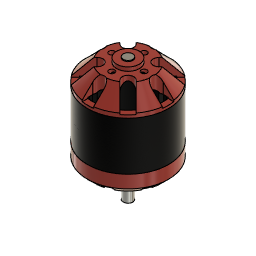
C4250-560KV (Autodesk Fusion 360 design; units mm, degrees)
Autodesk Fusion 360 part; units mm, degrees
sketch "Skizze1" plane through (0, 0, 0) normal (0, 0, 1) x (1, 0, 0)
  circle A0 centre (0, 0) radius 2.5
  dimension "d1" = 5
  constraint coincident A0.centre origin
  measures "d1" diameter of A0
extrude "Extrusion1" add sketch "Skizze1" against normal blind 0.5 makes body 1
sketch "Skizze2" plane through (0, 0, -0.5) normal (0, 0, -1) x (1, 0, 0)
  circle A0 centre (0, 0) radius 2.5
  circle A1 centre (0, 0) radius 5.95
  dimension "d4" = 11.9
  constraint coincident A0.centre A1.centre
  measures "d4" diameter of A1
extrude "Extrusion2" add sketch "Skizze2" along normal blind 2 separate body makes body 2
sketch "Skizze3" plane through (0, 0, -0.5) normal (0, 0, 1) x (-1, 0, 0)
  circle A0 centre (0, 0) radius 2.5
  circle A1 centre (0, 0) radius 5.95
sketch "Skizze4" plane through (0, 0, -2.5) normal (0, 0, -1) x (1, 0, 0)
  circle A0 centre (0, 0) radius 2.5
  circle A1 centre (0, 0) radius 5.95
  circle A2 centre (0, 0) radius 21.3
  dimension "d7" = 42.6
  constraint concentric A0 A2
  measures "d7" diameter of A2
extrude "Extrusion3" add sketch "Skizze4" along normal blind 46 separate body contours A2 makes body 3
sketch "Skizze5" plane through (0, 0, -2.5) normal (0, 0, 1) x (-1, 0, 0)
  circle A0 centre (0, 0) radius 5.95
  circle A1 centre (0, 0) radius 21.3
  circle A2 centre (0, 0) radius 12.75 construction
  dimension "d10" = 25.5
  constraint concentric A0 A2
  measures "d10" diameter of A2
chamfer "Fase1" distance 8.3 angle 45 1 edges at (-19.8586, 7.7024, -2.5) on bodies 3
sketch "Skizze6" plane through (0, 0, -2.5) normal (0, 0, 1) x (-1, 0, 0)
  circle A0 centre (8.5, 0) radius 1.5
  circle A1 centre (0, 8.5) radius 1.5
  circle A2 centre (-8.5, 0) radius 1.5
  circle A3 centre (0, -8.5) radius 1.5
  dimension "d13" = 3
  dimension "d15" = 360
  measures "d13" diameter of A0
extrude "Extrusion4" cut sketch "Skizze6" against normal blind 7 bodies 3
sketch "Skizze7" plane through (0, 0, -2.5) normal (0, 0, 1) x (-1, 0, 0)
  circle A0 centre (0, -8.5) radius 1.5
  circle A1 centre (8.5, 0) radius 1.5
  circle A2 centre (-8.5, 0) radius 1.5
  circle A3 centre (0, 8.5) radius 1.5
  circle A4 centre (0, 0) radius 5.95
  circle A5 centre (0, 0) radius 13
  line L0 (14.5681, -10.3255) -> (10.253, -6.0104)
  line L1 (10.3255, -14.5681) -> (6.0104, -10.253)
  arc A6 (10.253, -6.0104) -> (6.0104, -10.253) centre (8.1317, -8.1317) ccw
  line L2 (10.3255, -14.5681) -> (10.6437, -14.8863)
  line L3 (14.5681, -10.3255) -> (14.8863, -10.6437)
  arc A7 (10.6437, -14.8863) -> (14.8863, -10.6437) centre (0, 0) ccw
  arc A8 (14.8863, 10.6437) -> (10.6437, 14.8863) centre (0, 0) ccw
  line L4 (10.3255, 14.5681) -> (6.0104, 10.253)
  arc A9 (6.0104, 10.253) -> (10.253, 6.0104) centre (8.1317, 8.1317) ccw
  line L5 (14.5681, 10.3255) -> (10.253, 6.0104)
  line L6 (10.3255, 14.5681) -> (10.6437, 14.8863)
  arc A10 (-10.6437, 14.8863) -> (-14.8863, 10.6437) centre (0, 0) ccw
  line L7 (-14.5681, 10.3255) -> (-10.253, 6.0104)
  arc A11 (-10.253, 6.0104) -> (-6.0104, 10.253) centre (-8.1317, 8.1317) ccw
  line L8 (-10.3255, 14.5681) -> (-6.0104, 10.253)
  line L9 (-14.5681, 10.3255) -> (-14.8863, 10.6437)
  arc A12 (-14.8863, -10.6437) -> (-10.6437, -14.8863) centre (0, 0) ccw
  line L10 (-10.3255, -14.5681) -> (-6.0104, -10.253)
  arc A13 (-6.0104, -10.253) -> (-10.253, -6.0104) centre (-8.1317, -8.1317) ccw
  line L11 (-14.5681, -10.3255) -> (-10.253, -6.0104)
  line L12 (-10.3255, -14.5681) -> (-10.6437, -14.8863)
  line L13 (-14.5681, -10.3255) -> (-14.8863, -10.6437)
  line L14 (-10.3255, 14.5681) -> (-10.6437, 14.8863)
  line L15 (14.5681, 10.3255) -> (14.8863, 10.6437)
  line L16 (14.8863, -10.6437) -> (17.0326, -12.7899)
  line L17 (10.6437, -14.8863) -> (12.7899, -17.0326)
  arc A14 (12.7899, -17.0326) -> (17.0326, -12.7899) centre (0, 0) ccw
  line L18 (10.6437, 14.8863) -> (12.7899, 17.0326)
  arc A15 (17.0326, 12.7899) -> (12.7899, 17.0326) centre (0, 0) ccw
  line L19 (14.8863, 10.6437) -> (17.0326, 12.7899)
  line L20 (-14.8863, 10.6437) -> (-17.0326, 12.7899)
  arc A16 (-12.7899, 17.0326) -> (-17.0326, 12.7899) centre (0, 0) ccw
  line L21 (-10.6437, 14.8863) -> (-12.7899, 17.0326)
  line L22 (-10.6437, -14.8863) -> (-12.7899, -17.0326)
  arc A17 (-17.0326, -12.7899) -> (-12.7899, -17.0326) centre (0, 0) ccw
  line L23 (-14.8863, -10.6437) -> (-17.0326, -12.7899)
  dimension "d34" = 360
  dimension "d41" = 360
  constraint tangent L0 A6
  constraint tangent L1 A6
  constraint coincident A4.centre A5.centre
  constraint parallel L1 L2
  constraint parallel L0 L3
  constraint parallel L11 L13
  constraint concentric A7 A14
  constraint parallel L3 L16
  constraint parallel L2 L17
extrude "Extrusion5" cut sketch "Skizze7" against normal blind 9 contours A5 L4 A9 L5 | A5 A8 L4 L5 L6 L15 | A5 L0 L1 L2 L3 A7 | A5 L0 L1 A6 | A5 L7 A11 L8 | A5 A10 L7 L8 L9 L14 | A8 L18 A15 L19 | A5 A12 L10 L11 L12 L13 | A5 L10 A13 L11 | A7 L16 L17 A14 | A10 L20 A16 L21 | A12 L22 A17 L23 bodies 3
extrude "Extrusion6" cut sketch "Skizze7" against normal blind 15 contours A5 L4 A9 L5 | A5 A8 L4 L5 L6 L15 | A5 L0 L1 L2 L3 A7 | A5 L0 L1 A6 | A5 L7 A11 L8 | A5 A10 L7 L8 L9 L14 | A5 A12 L10 L11 L12 L13 | A5 L10 A13 L11 bodies 3
sketch "Skizze8" plane through (0, 0, -2.5) normal (0, 0, 1) x (-1, 0, 0)
  line L0 (-11.0656, -6.823) -> (-10.253, -6.0104)
  arc A0 (-6.0104, -10.253) -> (-10.253, -6.0104) centre (-8.1317, -8.1317) ccw
  line L1 (-6.0104, -10.253) -> (-6.823, -11.0656)
  arc A1 (-6.823, -11.0656) -> (6.823, -11.0656) centre (0, 0) ccw
  line L2 (6.823, -11.0656) -> (6.0104, -10.253)
  arc A2 (10.253, -6.0104) -> (6.0104, -10.253) centre (8.1317, -8.1317) ccw
  line L3 (10.253, -6.0104) -> (11.0656, -6.823)
  arc A3 (11.0656, -6.823) -> (11.0656, 6.823) centre (0, 0) ccw
  line L4 (11.0656, 6.823) -> (10.253, 6.0104)
  arc A4 (6.0104, 10.253) -> (10.253, 6.0104) centre (8.1317, 8.1317) ccw
  line L5 (6.0104, 10.253) -> (6.823, 11.0656)
  arc A5 (6.823, 11.0656) -> (-6.823, 11.0656) centre (0, 0) ccw
  line L6 (-6.823, 11.0656) -> (-6.0104, 10.253)
  arc A6 (-10.253, 6.0104) -> (-6.0104, 10.253) centre (-8.1317, 8.1317) ccw
  line L7 (-10.253, 6.0104) -> (-11.0656, 6.823)
  arc A7 (-11.0656, 6.823) -> (-11.0656, -6.823) centre (0, 0) ccw
  circle A8 centre (0, 0) radius 5.95
  circle A9 centre (0, 8.5) radius 1.5
  circle A10 centre (-8.5, 0) radius 1.5
  circle A11 centre (8.5, 0) radius 1.5
  circle A12 centre (0, -8.5) radius 1.5
  line L8 (-15.5, 0) -> (-15.5, -3) construction
  line L9 (-15.5, 0) -> (-15.5, 3) construction
  line L10 (-15.5, -3) -> (-18.0524, -3)
  line L11 (-18.0524, -3) -> (-21.0877, -3)
  line L12 (-15.5, 3) -> (-21.0877, 3)
  arc A13 (-21.0877, 3) -> (-21.0877, -3) centre (0, 0) ccw
  arc A14 (-18.0524, 3) -> (-18.0524, -3) centre (0, 0) ccw
  arc A15 (-15.5, -3) -> (-15.5, 3) centre (-15.5, 0) ccw
  arc A16 (3, -15.5) -> (-3, -15.5) centre (0, -15.5) ccw
  line L13 (3, -15.5) -> (3, -18.0524)
  line L14 (-3, -15.5) -> (-3, -21.0877)
  arc A17 (-3, -18.0524) -> (3, -18.0524) centre (0, 0) ccw
  arc A18 (-3, -21.0877) -> (3, -21.0877) centre (0, 0) ccw
  line L15 (3, -18.0524) -> (3, -21.0877)
  arc A19 (15.5, 3) -> (15.5, -3) centre (15.5, 0) ccw
  line L16 (15.5, 3) -> (18.0524, 3)
  line L17 (15.5, -3) -> (21.0877, -3)
  arc A20 (18.0524, -3) -> (18.0524, 3) centre (0, 0) ccw
  arc A21 (21.0877, -3) -> (21.0877, 3) centre (0, 0) ccw
  line L18 (18.0524, 3) -> (21.0877, 3)
  arc A22 (-3, 15.5) -> (3, 15.5) centre (0, 15.5) ccw
  line L19 (-3, 15.5) -> (-3, 18.0524)
  line L20 (3, 15.5) -> (3, 21.0877)
  arc A23 (3, 18.0524) -> (-3, 18.0524) centre (0, 0) ccw
  arc A24 (3, 21.0877) -> (-3, 21.0877) centre (0, 0) ccw
  line L21 (-3, 18.0524) -> (-3, 21.0877)
  dimension "d51" = 360
  constraint coincident L8.start L9.start
  constraint concentric A13 A14
  constraint tangent L10 A15
  constraint parallel L10 L11
  constraint tangent L12 A15
  constraint coincident L12 A14.start
extrude "Extrusion7" cut sketch "Skizze8" against normal blind 9 contours A7 L10 L12 A14 A15 | A7 A15 | L11 L12 A13 A14 | A1 A16 | A1 A16 L13 L14 A17 | L14 A17 A18 L15 | A5 A22 L19 L20 A23 | A5 A22 | L20 A23 A24 L21 | A3 A19 | A3 A19 L16 L17 A20 | L17 A20 A21 L18 bodies 3
extrude "Extrusion8" cut sketch "Skizze8" against normal blind 15 contours A7 L10 L12 A14 A15 | A7 A15 | A1 A16 | A1 A16 L13 L14 A17 | A5 A22 L19 L20 A23 | A5 A22 | A3 A19 | A3 A19 L16 L17 A20 bodies 3
extrude "Extrusion9" cut 1 faces at (16.0819, 1.3538, -48.5) along direction (0, 0, 1) blind 35.5 on bodies 3 bodies 3
sketch "Skizze9" plane through (0, 0, -13) normal (0, 0, -1) x (1, 0, 0)
  arc A0 (-3, -18.0524) -> (3, -18.0524) centre (0, 0) ccw
  line L0 (-3, -18.0524) -> (-3, -15.5)
  arc A1 (3, -15.5) -> (-3, -15.5) centre (0, -15.5) ccw
  line L1 (3, -15.5) -> (3, -18.0524)
  arc A2 (18.0524, -3) -> (18.0524, 3) centre (0, 0) ccw
  line L2 (18.0524, -3) -> (15.5, -3)
  arc A3 (15.5, 3) -> (15.5, -3) centre (15.5, 0) ccw
  line L3 (15.5, 3) -> (18.0524, 3)
  arc A4 (-18.0524, 3) -> (-18.0524, -3) centre (0, 0) ccw
  line L4 (-18.0524, 3) -> (-15.5, 3)
  arc A5 (-15.5, -3) -> (-15.5, 3) centre (-15.5, 0) ccw
  line L5 (-15.5, -3) -> (-18.0524, -3)
  arc A6 (3, 18.0524) -> (-3, 18.0524) centre (0, 0) ccw
  line L6 (3, 18.0524) -> (3, 15.5)
  arc A7 (-3, 15.5) -> (3, 15.5) centre (0, 15.5) ccw
  line L7 (-3, 15.5) -> (-3, 18.0524)
  arc A8 (14.8863, 10.6437) -> (10.6437, 14.8863) centre (0, 0) ccw
  line L8 (14.8863, 10.6437) -> (10.253, 6.0104)
  arc A9 (6.0104, 10.253) -> (10.253, 6.0104) centre (8.1317, 8.1317) ccw
  line L9 (6.0104, 10.253) -> (10.6437, 14.8863)
  arc A10 (10.6437, -14.8863) -> (14.8863, -10.6437) centre (0, 0) ccw
  line L10 (10.6437, -14.8863) -> (6.0104, -10.253)
  arc A11 (10.253, -6.0104) -> (6.0104, -10.253) centre (8.1317, -8.1317) ccw
  line L11 (10.253, -6.0104) -> (14.8863, -10.6437)
  arc A12 (-10.6437, 14.8863) -> (-14.8863, 10.6437) centre (0, 0) ccw
  line L12 (-10.6437, 14.8863) -> (-6.0104, 10.253)
  arc A13 (-10.253, 6.0104) -> (-6.0104, 10.253) centre (-8.1317, 8.1317) ccw
  line L13 (-10.253, 6.0104) -> (-14.8863, 10.6437)
  arc A14 (-14.8863, -10.6437) -> (-10.6437, -14.8863) centre (0, 0) ccw
  line L14 (-14.8863, -10.6437) -> (-10.253, -6.0104)
  arc A15 (-6.0104, -10.253) -> (-10.253, -6.0104) centre (-8.1317, -8.1317) ccw
  line L15 (-6.0104, -10.253) -> (-10.6437, -14.8863)
  circle A16 centre (0, 0) radius 5.95
  circle A17 centre (0, 0) radius 21.3
  circle A18 centre (0, 0) radius 12.5
  constraint concentric A0 A18
  constraint tangent A3 A18
sketch "Skizze10" plane through (0, 0, -13) normal (0, 0, -1) x (1, 0, 0)
  arc A0 (-3, -18.0524) -> (3, -18.0524) centre (0, 0) ccw
  line L0 (-3, -18.0524) -> (-3, -15.5)
  arc A1 (3, -15.5) -> (-3, -15.5) centre (0, -15.5) ccw
  line L1 (3, -15.5) -> (3, -18.0524)
  arc A2 (18.0524, -3) -> (18.0524, 3) centre (0, 0) ccw
  line L2 (18.0524, -3) -> (15.5, -3)
  arc A3 (15.5, 3) -> (15.5, -3) centre (15.5, 0) ccw
  line L3 (15.5, 3) -> (18.0524, 3)
  arc A4 (-18.0524, 3) -> (-18.0524, -3) centre (0, 0) ccw
  line L4 (-18.0524, 3) -> (-15.5, 3)
  arc A5 (-15.5, -3) -> (-15.5, 3) centre (-15.5, 0) ccw
  line L5 (-15.5, -3) -> (-18.0524, -3)
  arc A6 (3, 18.0524) -> (-3, 18.0524) centre (0, 0) ccw
  line L6 (3, 18.0524) -> (3, 15.5)
  arc A7 (-3, 15.5) -> (3, 15.5) centre (0, 15.5) ccw
  line L7 (-3, 15.5) -> (-3, 18.0524)
  arc A8 (14.8863, 10.6437) -> (10.6437, 14.8863) centre (0, 0) ccw
  line L8 (14.8863, 10.6437) -> (10.253, 6.0104)
  arc A9 (6.0104, 10.253) -> (10.253, 6.0104) centre (8.1317, 8.1317) ccw
  line L9 (6.0104, 10.253) -> (10.6437, 14.8863)
  arc A10 (10.6437, -14.8863) -> (14.8863, -10.6437) centre (0, 0) ccw
  line L10 (10.6437, -14.8863) -> (6.0104, -10.253)
  arc A11 (10.253, -6.0104) -> (6.0104, -10.253) centre (8.1317, -8.1317) ccw
  line L11 (10.253, -6.0104) -> (14.8863, -10.6437)
  arc A12 (-10.6437, 14.8863) -> (-14.8863, 10.6437) centre (0, 0) ccw
  line L12 (-10.6437, 14.8863) -> (-6.0104, 10.253)
  arc A13 (-10.253, 6.0104) -> (-6.0104, 10.253) centre (-8.1317, 8.1317) ccw
  line L13 (-10.253, 6.0104) -> (-14.8863, 10.6437)
  arc A14 (-14.8863, -10.6437) -> (-10.6437, -14.8863) centre (0, 0) ccw
  line L14 (-14.8863, -10.6437) -> (-10.253, -6.0104)
  arc A15 (-6.0104, -10.253) -> (-10.253, -6.0104) centre (-8.1317, -8.1317) ccw
  line L15 (-6.0104, -10.253) -> (-10.6437, -14.8863)
  circle A16 centre (0, 0) radius 5.95
  circle A17 centre (0, 0) radius 21.3
  circle A18 centre (0, 0) radius 18.3
  circle A19 centre (0, 0) radius 18.3
  constraint coincident A0.centre A2.centre
  constraint concentric A18 A19
extrude "Extrusion10" cut sketch "Skizze10" against normal blind 2 contours L0 A1 L1 L2 A3 L3 L4 A5 L5 L6 A7 L7 L8 A9 L9 L10 A11 L11 L12 A13 L13 L14 A15 L15 A18 A19 bodies 3
chamfer "Fase2" distance 8.5 angle 45 1 edges at (-5.5473, 2.1516, -11) on bodies 3
extrude "Extrusion11" add 1 faces at (3.1105, -20.0196, -13) along direction (0, 0, -1) blind 35.5 separate body on bodies 3 makes body 4
extrude "Extrusion12" cut 1 faces at (3.1105, -20.0196, -48.5) along direction (0, 0, 1) blind 10 on bodies 4 bodies 4
sketch "Skizze11" plane through (0, 0, -38.5) normal (0, 0, -1) x (1, 0, 0)
  circle A0 centre (0, 0) radius 21.3
  circle A1 centre (0, 0) radius 18.3
  circle A2 centre (0, 0) radius 21.3
  constraint concentric A0 A2
extrude "Extrusion13" add sketch "Skizze11" along normal blind 10 separate body contours A0 A2 | A1 makes body 5
sketch "Skizze12" plane through (0, 0, -48.5) normal (0, 0, -1) x (1, 0, 0)
  circle A0 centre (0, 0) radius 21.3
  circle A1 centre (8.8388, 8.8388) radius 1.5
  circle A2 centre (-8.8388, 8.8388) radius 1.5
  circle A3 centre (-8.8388, -8.8388) radius 1.5
  circle A4 centre (8.8388, -8.8388) radius 1.5
  circle A5 centre (0, 0) radius 6.75
  line L0 (0, 0) -> (0, -13) construction
  circle A6 centre (0, -13) radius 2
  circle A7 centre (0, 0) radius 20.8
  circle A8 centre (13, 0) radius 2
  circle A9 centre (-13, 0) radius 2
  line L1 (0, 0) -> (3.8268, 9.2388) construction
  circle A10 centre (3.8268, 9.2388) radius 2
  circle A11 centre (-3.8268, 9.2388) radius 2
  circle A12 centre (-9.2388, -3.8268) radius 2
  circle A13 centre (-13, 0) radius 2
  circle A14 centre (-9.2388, 3.8268) radius 2
  circle A15 centre (3.8268, -9.2388) radius 2
  circle A16 centre (0, -13) radius 2
  circle A17 centre (-3.8268, -9.2388) radius 2
  circle A18 centre (9.2388, 3.8268) radius 2
  circle A19 centre (13, 0) radius 2
  circle A20 centre (9.2388, -3.8268) radius 2
  line L2 (0, 0) -> (2, 0) construction
  line L3 (-1.9684, 9.9779) -> (-5.9293, 19.937)
  line L4 (0, 0) -> (-2, 0) construction
  line L5 (-5.6617, 8.443) -> (-9.9272, 18.2782)
  line L6 (-2, 13) -> (-2, 20.7036)
  line L7 (2, 13) -> (2, 20.7036)
  line L8 (1.9684, 9.9779) -> (5.9293, 19.937)
  line L9 (5.6617, 8.443) -> (9.9272, 18.2782)
  line L10 (-8.443, -5.6617) -> (-18.2782, -9.9272)
  line L11 (-9.9779, -1.9684) -> (-19.937, -5.9293)
  line L12 (-13, -2) -> (-20.7036, -2)
  line L13 (-13, 2) -> (-20.7036, 2)
  line L14 (-9.9779, 1.9684) -> (-19.937, 5.9293)
  line L15 (-8.443, 5.6617) -> (-18.2782, 9.9272)
  line L16 (5.6617, -8.443) -> (9.9272, -18.2782)
  line L17 (1.9684, -9.9779) -> (5.9293, -19.937)
  line L18 (2, -13) -> (2, -20.7036)
  line L19 (-2, -13) -> (-2, -20.7036)
  line L20 (-1.9684, -9.9779) -> (-5.9293, -19.937)
  line L21 (-5.6617, -8.443) -> (-9.9272, -18.2782)
  line L22 (8.443, 5.6617) -> (18.2782, 9.9272)
  line L23 (9.9779, 1.9684) -> (19.937, 5.9293)
  line L24 (13, 2) -> (20.7036, 2)
  line L25 (13, -2) -> (20.7036, -2)
  line L26 (9.9779, -1.9684) -> (19.937, -5.9293)
  line L27 (8.443, -5.6617) -> (18.2782, -9.9272)
  arc A21 (-2, 13) -> (2, 13) centre (0, 13) ccw
  circle A22 centre (0, 0) radius 18 construction
  dimension "d71" = 360
  dimension "d77" = 360
  dimension "d88" = 360
  dimension "d89" = 2
  dimension "d90" = 2
  dimension "d93" = 360
  dimension "d94" = 36
  constraint coincident A0.centre A5.centre
  constraint coincident L0.end A6.centre
  constraint coincident L1.end A10.centre
  constraint perpendicular L0 L2
  constraint coincident A11 L3.start
  constraint coincident A7 L3.end
  constraint tangent A11 L3
  constraint perpendicular L0 L4
  constraint coincident A11 L5.start
  constraint coincident A7 L5.end
  constraint tangent A11 L5
  constraint coincident A7 L6.end
  constraint tangent L6 A21
  constraint coincident A7 L7.end
  constraint tangent L7 A21
  constraint coincident A10 L8.start
  constraint coincident A7 L8.end
  constraint coincident A10 L9.start
  constraint coincident A7 L9.end
  constraint tangent A10 L9
  constraint concentric A7 A22
  measures "d89" distance of A0.centre L2.end
  measures "d90" distance of A0.centre L4.end
  measures "d94" diameter of A22
chamfer "Fase3" distance 3.3 angle 45 1 edges at (-19.8586, 7.7024, -48.5) on bodies 5
extrude "Extrusion14" cut sketch "Skizze12" against normal blind 1.5 contours A6 A16 | A6 A7 A16 L18 L19 | A7 A15 L16 L17 | A7 A17 L20 L21 | A15 | A17 | A7 A20 L26 L27 | A7 A12 L10 L11 | A20 | A12 | A7 A8 A19 L24 L25 | A7 A9 A13 L12 L13 | A8 A19 | A9 A13 | A7 A14 L14 L15 | A7 A18 L22 L23 | A14 | A18 | A7 A11 L3 L5 | A7 A10 L8 L9 | A11 | A10 | A7 L6 L7 A21 bodies 5
extrude "Extrusion15" cut 9 faces at (-4.8121, -12.2315, -47) (0.2226, -15.1629, -47) (4.8121, -12.2315, -47) (12.2315, -4.8121, -47) (15.1667, 0, -47) (12.2315, 4.8121, -47) (4.8121, 12.2315, -47) (-0.2226, 15.1629, -47) (-4.8121, 12.2315, -47) along direction (0, 0, 1) blind 5.7 on bodies 5 bodies 5
extrude "Extrusion16" cut sketch "Skizze12" against normal blind 7.3 contours A6 A16 | A6 A7 A16 L18 L19 | A7 A15 L16 L17 | A7 A17 L20 L21 | A15 | A17 | A7 A12 L10 L11 | A12 | A7 A9 A13 L12 L13 | A9 A13 | A7 A14 L14 L15 | A14 | A7 A11 L3 L5 | A7 A10 L8 L9 | A11 | A10 | A7 L6 L7 A21 bodies 5
extrude "Extrusion17" cut 9 faces at (4.9765, 12.6327, -41.2) (-0.2225, 15.5964, -41.2) (-4.9765, 12.6327, -41.2) (-12.6327, 4.9765, -41.2) (-15.5964, 0.2225, -41.2) (-12.6327, -4.9765, -41.2) (-4.9765, -12.6327, -41.2) (-0.2225, -15.5964, -41.2) (4.9765, -12.6327, -41.2) along direction (0, 0, 1) blind 15 on bodies 5 bodies 4 5
extrude "Extrusion18" cut sketch "Skizze12" against normal blind 15 contours A1 | A2 | A3 | A4 bodies 5
extrude "Extrusion19" cut sketch "Skizze12" against normal blind 1.8 contours A5 bodies 5
sketch "Skizze13" plane through (0, 0, -46.7) normal (0, 0, -1) x (1, 0, 0)
  circle A0 centre (0, 0) radius 6.75
  circle A1 centre (0, 0) radius 2.5
  dimension "d108" = 5
  constraint concentric A0 A1
  measures "d108" diameter of A1
extrude "Extrusion20" add sketch "Skizze13" along normal blind 20 separate body contours A1 makes body 6
extrude "Extrusion21" cut 1 faces at (-0.8863, -0.2321, -66.7) along direction (0, 0, 1) blind 1.7 on bodies 6 bodies 6
equation "d56 = -37 mm + 1.5 mm"
equation "d61 = 46 mm - 10.5 mm"
equation "d98 = -7.2 mm + 1.5 mm"
